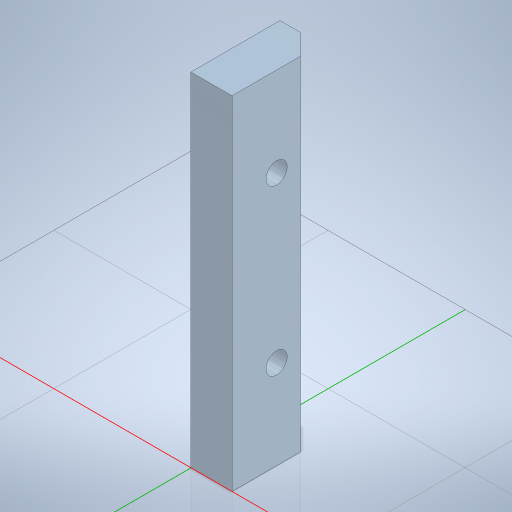
# Autodesk Inventor part: Flach_Alu
Saved by Autodesk Inventor 2024 (Build 280153000, 153)
## iProperties
Created: 2024-04-02
Part Number: Flach_Alu
Material: Aluminium 6061
Document SubType Name: Modeling
Designer: ffogue
Density: 2.7 g/cm^3
Appearance: Stahlblau
Author: ffogue
Autodesk Inventor part; units mm, degrees
ref_plane "YZ Plane" through (0, 0, 0) normal (1, 0, 0) x (0, 1, 0)
ref_plane "XZ Plane" through (0, 0, 0) normal (0, 1, 0) x (-1, 0, 0)
ref_plane "XY Plane" through (0, 0, 0) normal (0, 0, 1) x (1, 0, 0)
sketch "Skizze1" plane through (0, 0, 0) normal (0, 0, 1) x (1, 0, 0)
  line L0 (0, 0) -> (0, 13)
  line L1 (0, 13) -> (3, 13)
  line L2 (3, 13) -> (6, 10)
  line L3 (6, 10) -> (6, 0)
  line L4 (6, 0) -> (0, 0)
  dimension "d0" = 6
  dimension "d1" = 13
  dimension "d2" = 3
  dimension "d3" = 45
  constraints: 10 end point, 2 perpendicular, 1 parallel, 1 vertical
  measures "d0" distance between parallel lines of L3 L0
  measures "d1" distance between parallel lines of L4 L1
  measures "d2" horizontal distance of L2.end L1.end
  measures "d3" angle of L2 L3
extrude "Extrusion1" add sketch "Skizze1" along normal blind 50
sketch "Skizze2" plane through (0, 0, 0) normal (-1, 0, 0) x (0, 0, 1)
  line L0 (0, 13) -> (0, 0) projected
  point P0 (13, 6.5)
  point P1 (37, 6.5)
  point P2 (0, 6.5)
  point P3 (0, 6.5)
  dimension "d13" = 24
  dimension "d14" = 13
  constraints: 2 horizontal alignment, 2 midpoint
  measures "d13" distance of point (37, 6.5) point (13, 6.5)
  measures "d14" distance of point (13, 6.5) point (0, 6.5)
hole "Bohrung1" at (0, 6.5, 13) at (0, 6.5, 37) direction (1, 0, 0) diameter 3.1 end through all
